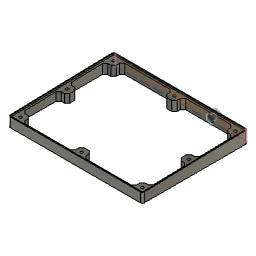
case (Autodesk Fusion 360 design; units mm, degrees)
Autodesk Fusion 360 part; units mm, degrees
sketch "Sketch1" plane through (0, 0, 0) normal (0, 0, 1) x (1, 0, 0)
  line L0 (0, 0) -> (294.692, 0)
  line L1 (294.692, 0) -> (294.692, 230.4)
  line L2 (294.692, 230.4) -> (0, 230.4)
  line L3 (0, 230.4) -> (0, 0)
  line L4 (-2, 232.4) -> (296.692, 232.4)
  line L5 (296.692, 232.4) -> (296.692, -2)
  line L6 (296.692, -2) -> (-2, -2)
  line L7 (-2, -2) -> (-2, 232.4)
  line L8 (0, 230.4) -> (23, 230.4)
  line L9 (23, 230.4) -> (23, 207.4)
  line L10 (23, 207.4) -> (0, 207.4)
  line L11 (0, 207.4) -> (0, 230.4)
  line L12 (294.692, 230.4) -> (271.692, 230.4)
  line L13 (271.692, 230.4) -> (271.692, 207.4)
  line L14 (271.692, 207.4) -> (294.692, 207.4)
  line L15 (294.692, 207.4) -> (294.692, 230.4)
  line L16 (0, 0) -> (23, 0)
  line L17 (23, 0) -> (23, 23)
  line L18 (23, 23) -> (0, 23)
  line L19 (0, 23) -> (0, 0)
  line L20 (294.692, 0) -> (271.692, 0)
  line L21 (271.692, 0) -> (271.692, 23)
  line L22 (271.692, 23) -> (294.692, 23)
  line L23 (294.692, 23) -> (294.692, 0)
  line L24 (0, 0) -> (294.692, 230.4) construction
  line L25 (0, 230.4) -> (294.692, 0) construction
  line L26 (147.346, 230.4) -> (147.346, 0) construction
  line L27 (0, 115.2) -> (294.692, 115.2) construction
  line L28 (135.846, 230.4) -> (158.846, 230.4)
  line L29 (158.846, 230.4) -> (158.846, 207.4)
  line L30 (158.846, 207.4) -> (135.846, 207.4)
  line L31 (135.846, 207.4) -> (135.846, 230.4)
  line L32 (135.846, 230.4) -> (158.846, 207.4) construction
  line L33 (135.846, 207.4) -> (158.846, 230.4) construction
  circle A0 centre (147.346, 218.9) radius 3
  line L34 (0, 207.4) -> (23, 230.4) construction
  line L35 (23, 207.4) -> (0, 230.4) construction
  circle A1 centre (11.5, 218.9) radius 3
  line L36 (0, 23) -> (23, 0) construction
  line L37 (23, 23) -> (0, 0) construction
  circle A2 centre (11.5, 11.5) radius 3
  line L38 (271.692, 0) -> (294.692, 23) construction
  line L39 (271.692, 23) -> (294.692, 0) construction
  line L40 (294.692, 230.4) -> (271.692, 207.4) construction
  line L41 (271.692, 230.4) -> (294.692, 207.4) construction
  circle A3 centre (283.192, 218.9) radius 3
  circle A4 centre (283.192, 11.5) radius 3
  line L42 (135.846, 0) -> (158.846, 0)
  line L43 (158.846, 0) -> (158.846, 23)
  line L44 (158.846, 23) -> (135.846, 23)
  line L45 (135.846, 23) -> (135.846, 0)
  line L46 (0, 126.7) -> (23, 126.7)
  line L47 (23, 126.7) -> (23, 103.7)
  line L48 (23, 103.7) -> (0, 103.7)
  line L49 (0, 103.7) -> (0, 126.7)
  line L50 (294.692, 126.7) -> (271.692, 126.7)
  line L51 (271.692, 126.7) -> (271.692, 103.7)
  line L52 (271.692, 103.7) -> (294.692, 103.7)
  line L53 (294.692, 103.7) -> (294.692, 126.7)
  line L54 (135.846, 0) -> (158.846, 23) construction
  line L55 (135.846, 23) -> (158.846, 0) construction
  line L56 (294.692, 126.7) -> (271.692, 103.7) construction
  line L57 (271.692, 126.7) -> (294.692, 103.7) construction
  line L58 (0, 103.7) -> (23, 126.7) construction
  line L59 (0, 126.7) -> (23, 103.7) construction
  circle A5 centre (11.5, 115.2) radius 3
  circle A6 centre (147.346, 11.5) radius 3
  circle A7 centre (283.192, 115.2) radius 3
  line L60 (23, 230.4) -> (135.846, 230.4)
  line L61 (135.846, 230.4) -> (135.846, 226.4)
  line L62 (135.846, 226.4) -> (23, 226.4)
  line L63 (23, 226.4) -> (23, 230.4)
  line L64 (0, 207.4) -> (4, 207.4)
  line L65 (4, 207.4) -> (4, 126.7)
  line L66 (4, 126.7) -> (0, 126.7)
  line L67 (0, 126.7) -> (0, 207.4)
  line L68 (0, 103.7) -> (4, 103.7)
  line L69 (4, 103.7) -> (4, 23)
  line L70 (4, 23) -> (0, 23)
  line L71 (0, 23) -> (0, 103.7)
  line L72 (23, 0) -> (135.846, 0)
  line L73 (135.846, 0) -> (135.846, 4)
  line L74 (135.846, 4) -> (23, 4)
  line L75 (23, 4) -> (23, 0)
  line L76 (158.846, 0) -> (271.692, 0)
  line L77 (271.692, 0) -> (271.692, 4)
  line L78 (271.692, 4) -> (158.846, 4)
  line L79 (158.846, 4) -> (158.846, 0)
  line L80 (294.692, 23) -> (290.692, 23)
  line L81 (290.692, 23) -> (290.692, 103.7)
  line L82 (290.692, 103.7) -> (294.692, 103.7)
  line L83 (294.692, 103.7) -> (294.692, 23)
  line L84 (294.692, 126.7) -> (290.692, 126.7)
  line L85 (290.692, 126.7) -> (290.692, 207.4)
  line L86 (290.692, 207.4) -> (294.692, 207.4)
  line L87 (294.692, 207.4) -> (294.692, 126.7)
  line L88 (158.846, 230.4) -> (271.692, 230.4)
  line L89 (271.692, 230.4) -> (271.692, 226.4)
  line L90 (271.692, 226.4) -> (158.846, 226.4)
  line L91 (158.846, 226.4) -> (158.846, 230.4)
  dimension "d1" = 294.692
  dimension "d2" = 230.4
  dimension "d3" = 2
  dimension "d4" = 2
  dimension "d5" = 2
  dimension "d6" = 2
  dimension "d7" = 23
  dimension "d8" = 23
  dimension "d12" = 23
  dimension "d13" = 23
  dimension "d17" = 23
  dimension "d18" = 23
  dimension "d22" = 23
  dimension "d23" = 23
  dimension "d27" = 23
  dimension "d28" = 23
  dimension "d29" = 6
  dimension "d30" = 6
  dimension "d31" = 6
  dimension "d32" = 6
  dimension "d33" = 6
  dimension "d34" = 23
  dimension "d35" = 23
  dimension "d36" = 23
  dimension "d37" = 23
  dimension "d38" = 23
  dimension "d39" = 23
  dimension "d40" = 6
  dimension "d41" = 6
  dimension "d42" = 6
  dimension "d43" = 4
  dimension "d44" = 4
  dimension "d45" = 4
  dimension "d46" = 4
  dimension "d47" = 4
  dimension "d48" = 4
  dimension "d49" = 4
  dimension "d50" = 4
  constraint horizontal L0
  constraint vertical L1
  constraint horizontal L2
  constraint vertical L3
  constraint coincident L0.start L3.end
  constraint horizontal L4
  constraint vertical L5
  constraint horizontal L6
  constraint vertical L7
  constraint horizontal L8
  constraint vertical L9
  constraint horizontal L10
  constraint vertical L11
  constraint horizontal L12
  constraint vertical L13
  constraint horizontal L14
  constraint vertical L15
  constraint horizontal L16
  constraint vertical L17
  constraint horizontal L18
  constraint vertical L19
  constraint horizontal L20
  constraint vertical L21
  constraint horizontal L22
  constraint vertical L23
  constraint midpoint L2 L26.start
  constraint midpoint L0 L26.end
  constraint midpoint L3 L27.start
  constraint midpoint L1 L27.end
  constraint horizontal L28
  constraint vertical L29
  constraint horizontal L30
  constraint vertical L31
  constraint coincident L2 L28.start
  constraint symmetric L26 L29 L31
  constraint midpoint L33 A0.centre
  constraint midpoint L35 A1.centre
  constraint midpoint L36 A2.centre
  constraint midpoint L40 A3.centre
  constraint midpoint L38 A4.centre
  constraint horizontal L42
  constraint vertical L43
  constraint horizontal L44
  constraint vertical L45
  constraint coincident L0 L42.start
  constraint symmetric L26 L43 L45
  constraint horizontal L46
  constraint vertical L47
  constraint horizontal L48
  constraint vertical L49
  constraint coincident L3 L46.start
  constraint symmetric L27 L46 L48
  constraint horizontal L50
  constraint vertical L51
  constraint horizontal L52
  constraint vertical L53
  constraint coincident L1 L50.start
  constraint symmetric L27 L50 L52
  constraint midpoint L58 A5.centre
  constraint midpoint L54 A6.centre
  constraint midpoint L56 A7.centre
  constraint horizontal L60
  constraint vertical L61
  constraint horizontal L62
  constraint vertical L63
  constraint horizontal L64
  constraint vertical L65
  constraint horizontal L66
  constraint vertical L67
  constraint horizontal L68
  constraint vertical L69
  constraint horizontal L70
  constraint vertical L71
  constraint horizontal L72
  constraint vertical L73
  constraint horizontal L74
  constraint vertical L75
  constraint horizontal L76
  constraint vertical L77
  constraint horizontal L78
  constraint vertical L79
  constraint horizontal L80
  constraint vertical L81
  constraint horizontal L82
  constraint vertical L83
  constraint horizontal L84
  constraint vertical L85
  constraint horizontal L86
  constraint vertical L87
  constraint horizontal L88
  constraint vertical L89
  constraint horizontal L90
  constraint vertical L91
  measures "d1" distance of L0.start L0.end
  measures "d2" distance of L0.start L2.end
  measures "d3" distance of L2 L4
  measures "d4" distance of L1 L5
  measures "d5" distance of L0 L6
  measures "d6" distance of L3 L7
  measures "d7" distance of L2.end L8.end
  measures "d8" distance of L2.end L10.end
  measures "d12" distance of L1.end L12.end
  measures "d13" distance of L1.end L14.end
  measures "d17" distance of L0.start L16.end
  measures "d18" distance of L0.start L18.end
  measures "d22" distance of L0.end L20.end
  measures "d23" distance of L0.end L22.end
  measures "d27" distance of L28.start L28.end
  measures "d28" distance of L28.start L30.end
  measures "d29" diameter of A0
  measures "d30" diameter of A1
  measures "d31" diameter of A2
  measures "d32" diameter of A3
  measures "d33" diameter of A4
  measures "d34" distance of L42.start L42.end
  measures "d35" distance of L42.start L44.end
  measures "d36" distance of L46.start L46.end
  measures "d37" distance of L46.start L48.end
  measures "d38" distance of L50.start L50.end
  measures "d39" distance of L50.start L52.end
  measures "d40" diameter of A5
  measures "d41" diameter of A6
  measures "d42" diameter of A7
  measures "d43" distance of L8.end L62.end
  measures "d44" distance of L10.end L64.end
  measures "d45" distance of L48.end L68.end
  measures "d46" distance of L16.end L74.end
  measures "d47" distance of L42.end L78.end
  measures "d48" distance of L22.end L80.end
  measures "d49" distance of L50.start L84.end
  measures "d50" distance of L28.end L90.end
extrude "Extrude1" add sketch "Sketch1" along normal blind 22 contours L0 L3 L16 L17 L18 L19 L70 L75 | L0 L17 L45 L72 L73 L74 L75 | L3 L18 L48 L68 L69 L70 L71 | L0 L42 L43 L44 L45 L73 L79 | L3 L46 L47 L48 L49 L66 L68 | L0 L21 L43 L76 L77 L78 L79 | L3 L10 L46 L64 L65 L66 L67 | L0 L1 L20 L21 L22 L23 L77 L80 | L2 L3 L8 L9 L10 L11 L63 L64 | L1 L22 L52 L80 L81 L82 L83 | L2 L9 L31 L60 L61 L62 L63 | L1 L50 L51 L52 L53 L82 L84 | L2 L28 L29 L30 L31 L61 L91 | L1 L14 L50 L84 L85 L86 L87 | L2 L13 L29 L88 L89 L90 L91 | L1 L2 L12 L13 L14 L15 L86 L89 | L4 L5 L6 L7 makes body 1
sketch "Sketch2" plane through (0, 0, 22) normal (0, 0, 1) x (-1, 0, 0)
  line L0 (-271.692, -226.4) -> (-271.692, -207.4)
  line L1 (-271.692, -207.4) -> (-290.692, -207.4)
  line L2 (-290.692, -207.4) -> (-290.692, -126.7)
  line L3 (-290.692, -126.7) -> (-271.692, -126.7)
  line L4 (-271.692, -126.7) -> (-271.692, -103.7)
  line L5 (-271.692, -103.7) -> (-290.692, -103.7)
  line L6 (-290.692, -103.7) -> (-290.692, -23)
  line L7 (-290.692, -23) -> (-271.692, -23)
  line L8 (-271.692, -23) -> (-271.692, -4)
  line L9 (-271.692, -4) -> (-158.846, -4)
  line L10 (-158.846, -4) -> (-158.846, -23)
  line L11 (-158.846, -23) -> (-135.846, -23)
  line L12 (-135.846, -23) -> (-135.846, -4)
  line L13 (-135.846, -4) -> (-23, -4)
  line L14 (-23, -4) -> (-23, -23)
  line L15 (-23, -23) -> (-4, -23)
  line L16 (-4, -23) -> (-4, -103.7)
  line L17 (-4, -103.7) -> (-23, -103.7)
  line L18 (-23, -103.7) -> (-23, -126.7)
  line L19 (-23, -126.7) -> (-4, -126.7)
  line L20 (-4, -126.7) -> (-4, -207.4)
  line L21 (-4, -207.4) -> (-23, -207.4)
  line L22 (-23, -207.4) -> (-23, -226.4)
  line L23 (-23, -226.4) -> (-135.846, -226.4)
  line L24 (-135.846, -226.4) -> (-135.846, -207.4)
  line L25 (-135.846, -207.4) -> (-158.846, -207.4)
  line L26 (-158.846, -207.4) -> (-158.846, -226.4)
  line L27 (-158.846, -226.4) -> (-271.692, -226.4)
  circle A0 centre (-147.346, -11.5) radius 3
  circle A1 centre (-283.192, -11.5) radius 3
  circle A2 centre (-11.5, -115.2) radius 3
  circle A3 centre (-283.192, -115.2) radius 3
  circle A4 centre (-283.192, -218.9) radius 3
  circle A5 centre (-11.5, -11.5) radius 3
  circle A6 centre (-147.346, -218.9) radius 3
  circle A7 centre (-11.5, -218.9) radius 3
  line L28 (2, 2) -> (-296.692, 2)
  line L29 (-296.692, 2) -> (-296.692, -232.4)
  line L30 (-296.692, -232.4) -> (2, -232.4)
  line L31 (2, -232.4) -> (2, 2)
  line L32 (0, -230.4) -> (-294.692, -230.4)
  line L33 (-294.692, -230.4) -> (-294.692, 0)
  line L34 (-294.692, 0) -> (0, 0)
  line L35 (0, 0) -> (0, -230.4)
  dimension "d53" = 2
  dimension "d54" = 2
  dimension "d55" = 2
  dimension "d56" = 2
  constraint horizontal L32
  constraint vertical L33
  constraint horizontal L34
  constraint vertical L35
  measures "d53" distance of L31 L35
  measures "d54" distance of L30 L32
  measures "d55" distance of L29 L33
  measures "d56" distance of L28 L34
chamfer "Chamfer1" distance 6 angle 45 28 edges at (271.692, 4, 11) (271.692, 23, 11) (290.692, 23, 11) (290.692, 103.7, 11) (271.692, 103.7, 11) (271.692, 126.7, 11) (290.692, 126.7, 11) (135.846, 4, 11) (158.846, 4, 11) (135.846, 23, 11) (158.846, 23, 11) (23, 4, 11) (23, 23, 11) (4, 23, 11) (4, 103.7, 11) (4, 126.7, 11) (23, 126.7, 11) (23, 103.7, 11) (4, 207.4, 11) (23, 226.4, 11) (23, 207.4, 11) (135.846, 226.4, 11) (135.846, 207.4, 11) (158.846, 226.4, 11) (158.846, 207.4, 11) (271.692, 226.4, 11) (271.692, 207.4, 11) (290.692, 207.4, 11) on bodies 1
sketch "Sketch3" plane through (-2, 0, 0) normal (-1, 0, 0) x (0, -1, 0)
  line L0 (-232.4, 0) -> (2, 0)
  line L1 (2, 0) -> (2, 22)
  line L2 (2, 22) -> (-232.4, 22)
  line L3 (-232.4, 22) -> (-232.4, 0)
  line L4 (2, 0) -> (2, 16)
  line L5 (2, 16) -> (-232.4, 22)
  dimension "d62" = 16
  constraint coincident L0.end L1.start
  constraint perpendicular L0 L4
  constraint coincident L2.end L3.start
  measures "d62" distance of L0.end L4.end
extrude "Extrude4" cut sketch "Sketch3" against normal through all contours L1 L2 L5 bodies 1
extrude "Extrude5" add sketch "Sketch2" along normal blind 3 separate body contours L28 L29 L30 L31 makes body 2
extrude "Extrude6" add sketch "Sketch2" against normal through all of body 1 contours L28 L29 L30 L31 bodies 1 2
sketch "Sketch4" plane through (-2, 0, 0) normal (-1, 0, 0) x (0, -1, 0)
  line L0 (-232.4, 25) -> (-232.4, 0)
  line L1 (-232.4, 0) -> (2, 0)
  line L2 (2, 0) -> (2, 25)
  line L3 (2, 25) -> (-232.4, 25)
  line L4 (2, 0) -> (2, 19)
  line L5 (2, 19) -> (-232.4, 25)
  dimension "d67" = 19
  constraint coincident L1.end L2.start
  constraint perpendicular L1 L4
  constraint coincident L0.start L3.end
  measures "d67" distance of L1.end L4.end
extrude "Extrude7" cut sketch "Sketch4" against normal through all contours L2 L3 L5 bodies 1
extrude "Extrude8" add sketch "Sketch1" against normal blind 2 contours L4 L5 L6 L7 bodies 1
fillet "Fillet1" radius 4 4 edges at (-2, 232.4, 11.5) (-2, -2, 8.5) (296.692, -2, 8.5) (296.692, 232.4, 11.5) on bodies 1
fillet "Fillet2" radius 2 4 edges at (0, 230.4, 23.4488) (294.692, 230.4, 23.4488) (294.692, 0, 17.5512) (0, 0, 17.5512) on bodies 1
fillet "Fillet3" radius 2 4 edges at (0, 0, -1) (294.692, 0, -1) (294.692, 230.4, -1) (0, 230.4, -1) on bodies 1
sketch "Sketch5" plane through (0, 232.4, 0) normal (0, 1, 0) x (-1, 0, 0)
  line L0 (-2, 25) -> (-292.692, 25)
  line L1 (-292.692, -2) -> (-2, -2)
  line L2 (-294.692, 22) -> (0, 22) construction
  line L3 (0, 22) -> (0, 0) construction
  line L4 (0, 0) -> (-294.692, 0) construction
  line L5 (-294.692, 0) -> (-294.692, 22) construction
  line L6 (-294.692, 22) -> (0, 0) construction
  line L7 (0, 22) -> (-294.692, 0) construction
  line L8 (-147.346, 22) -> (-147.346, 0) construction
  line L9 (-294.692, 11) -> (0, 11) construction
  line L10 (-294.692, 0) -> (-147.346, 22) construction
  line L11 (-147.346, 0) -> (-294.692, 22) construction
  circle A0 centre (-221.019, 11) radius 6.3
  line L12 (-292.692, 25) -> (-292.692, -2)
  line L13 (-2, -2) -> (-2, 25)
  dimension "d77" = 3
  dimension "d79" = 2
  dimension "d81" = 12.6
  constraint horizontal L2
  constraint vertical L3
  constraint horizontal L4
  constraint vertical L5
  constraint midpoint L2 L8.start
  constraint midpoint L4 L8.end
  constraint midpoint L5 L9.start
  constraint midpoint L3 L9.end
  constraint midpoint L10 A0.centre
  measures "d77" distance of L0 L2
  measures "d79" distance of L1 L4
  measures "d81" diameter of A0
extrude "Extrude10" cut sketch "Sketch5" against normal blind 6 contours A0 bodies 1
sketch "Sketch7" plane through (0, 226.4, 0) normal (0, -1, 0) x (1, 0, 0)
  circle A0 centre (221.019, 11) radius 6.3
  line L0 (265.692, 21.8464) -> (164.846, 21.8464)
  line L1 (164.846, 21.8464) -> (164.846, 0)
  line L2 (164.846, 0) -> (265.692, 0)
  line L3 (265.692, 0) -> (265.692, 21.8464)
  circle A1 centre (221.019, 11) radius 6.8
  dimension "d89" = 13.6
  constraint concentric A0 A1
  measures "d89" diameter of A1
extrude "Extrude11" cut sketch "Sketch7" against normal blind 4 contours A1 bodies 1
equation "d67 = 16 mm + 3 mm"
